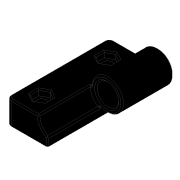
# Autodesk Inventor part: hing-leftSide
Saved by Autodesk Inventor 2015 (Build 190159000, 159)
## iProperties
Created: 2018-06-11
Part Number: hing-leftSide
Material: Generic
Document SubType Name: Modeling
Designer: Ghassan Yusuf
Density: 1 g/cm^3
Appearance: Default(2)
Author: Ghassan Yusuf
Autodesk Inventor part; units mm, degrees
ref_plane "YZ Plane" through (0, 0, 0) normal (1, 0, 0) x (0, 1, 0)
ref_plane "XZ Plane" through (0, 0, 0) normal (0, 1, 0) x (-1, 0, 0)
ref_plane "XY Plane" through (0, 0, 0) normal (0, 0, 1) x (1, 0, 0)
sketch "Sketch1" plane through (0, 0, 0) normal (0, 0, 1) x (1, 0, 0)
  line L0 (-16, 20) -> (0, 20)
  line L1 (0, 20) -> (0, -20)
  line L2 (0, -20) -> (-16, -20)
  line L3 (-16, -20) -> (-16, 20)
  circle A0 centre (-9.5, 12.75) radius 1.75
  circle A1 centre (-9.5, -12.75) radius 1.75
  point P0 (0, 0)
  point P1 (0, 0)
  dimension "d0" = 16
  dimension "d1" = 40
  dimension "d2" = 3.5
  dimension "d3" = 25.5
  dimension "d4" = 12.75
  dimension "d5" = 6.5
  constraints: 8 end point, 2 centre point, 2 midpoint, 2 parallel, 1 coincident, 1 equal radius, 1 horizontal, 1 perpendicular, 1 vertical alignment
  measures "d0" distance of L1.end L2.end
  measures "d1" distance of L0.end L1.end
  measures "d2" diameter of A0
  measures "d3" distance of A1.centre A0.centre
  measures "d4" vertical distance of point (0, 0) A0.centre
  measures "d5" distance from line of L3 A0.centre
extrude "Extrusion1" add sketch "Sketch1" along normal blind 9
sketch "Sketch2" plane through (0, 0, 0) normal (0, 1, 0) x (-1, 0, 0)
  circle A0 centre (-3, 9) radius 6
  line L0 (16, 9) -> (0, 9) projected
  line L1 (0, 0) -> (0, 9) projected
  circle A1 centre (-3, 9) radius 6.5
  dimension "d8" = 12
  dimension "d9" = 3
  dimension "d12" = 0.5
  constraints: 2 centre point, 1 point on line
  measures "d8" diameter of A0
  measures "d9" distance from line of L1 A0.centre
  measures "d12" radial gap between concentric circles of A0 A1
extrude "Extrusion2" add sketch "Sketch2" along normal blind 20 contours L0 L1 A0 | A0 L1 L0
extrude "Extrusion3" cut sketch "Sketch2" against normal blind 20
hole "Hole1" at (3, 0, 9) direction (0, 1, 0) diameter 8.4 end through all
fillet "Fillet4" radius 2 2 edges at (-16, -20, 4.5) (-16, 20, 4.5)
fillet "Fillet5" radius 0.34 2 edges at (0, 10, 3.8038) (-3, 10, 9)
chamfer "Chamfer1" distance 0.5 angle 45 11 edges at (0, 20, 1.6225) (0.1568, 20, 3.5314) (8.1398, 20, 12.0956) (-3.097, 20, 9.0932) (-8.6654, 20, 9) (-15.4142, 19.4142, 9) (-16, 0, 9) (-15.4142, -19.4142, 9) (-8.75, -20, 9) (0, -20, 1.6169) (-2.5565, -20, 5.6273)
chamfer "Chamfer2" distance 0.5 angle 45 2 edges at (-3.5, -9.75, 9) (0, -9.75, 3.2337)
chamfer "Chamfer3" distance 0.5 angle 45 7 edges at (8.1398, 0, 12.0956) (-3.097, 0, 9.0932) (-3.6654, 0, 9) (0.1568, 0, 3.5314) (0, 0, 2.9894) (3, 0, 13.2) (3, 20, 13.2)
sketch "Sketch3" plane through (0, 0, 9) normal (0, 0, 1) x (1, 0, 0)
  circle A0 centre (-9.5, 12.75) radius 1.75 projected
  line L0 (-9.5, 9.5168) -> (-12.3, 11.1334)
  line L1 (-12.3, 11.1334) -> (-12.3, 14.3666)
  line L2 (-12.3, 14.3666) -> (-9.5, 15.9832)
  line L3 (-9.5, 15.9832) -> (-6.7, 14.3666)
  line L4 (-6.7, 14.3666) -> (-6.7, 11.1334)
  line L5 (-6.7, 11.1334) -> (-9.5, 9.5168)
  circle A1 centre (-9.5, -12.75) radius 1.75 projected
  line L6 (-9.5, -9.5168) -> (-6.7, -11.1334)
  line L7 (-6.7, -11.1334) -> (-6.7, -14.3666)
  line L8 (-6.7, -14.3666) -> (-9.5, -15.9832)
  line L9 (-9.5, -15.9832) -> (-12.3, -14.3666)
  line L10 (-12.3, -14.3666) -> (-12.3, -11.1334)
  line L11 (-12.3, -11.1334) -> (-9.5, -9.5168)
  line L12 (-16, 18) -> (-16, -18) projected
  point P0 (0, 0)
  dimension "d38" = 5.6
  constraints: 24 end point, 2 coincident, 2 parallel, 1 collinear, 26 other
  measures "d38" distance between parallel lines of L4 L1
extrude "Extrusion4" cut sketch "Sketch3" against normal blind 2.3 contours A0 | L0 L1 L2 L3 L4 L5 | A1 | L6 L7 L8 L9 L10 L11
chamfer "Chamfer4" distance 0.5 angle 45 12 edges at (-10.9, 15.1749, 9) (-8.1, 15.1749, 9) (-12.3, 12.75, 9) (-10.9, 10.3251, 9) (-8.1, 10.3251, 9) (-6.7, 12.75, 9) (-12.3, -12.75, 9) (-10.9, -10.3251, 9) (-8.1, -10.3251, 9) (-6.7, -12.75, 9) (-8.1, -15.1749, 9) (-10.9, -15.1749, 9)
equation "\"d4\" = 0.5 * d3"
equation "\"d9\" = 0.25 * d8"
body "Solid1"
